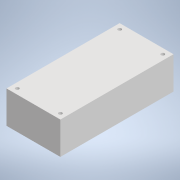
# Autodesk Inventor part: LPS_board
Saved by Autodesk Inventor 2022 (Build 260153000, 153)
## iProperties
Created: 2024-07-06
Part Number: LPS_board
Material: Типовые
Document SubType Name: Modeling
Designer: Капустяник Андрей
Density: 1 g/cm^3
Appearance: По умолчанию
Author: Капустяник Андрей
Autodesk Inventor part; units mm, degrees
ref_plane "YZ Plane" through (0, 0, 0) normal (1, 0, 0) x (0, 1, 0)
ref_plane "XZ Plane" through (0, 0, 0) normal (0, 1, 0) x (-1, 0, 0)
ref_plane "XY Plane" through (0, 0, 0) normal (0, 0, 1) x (1, 0, 0)
sketch "Эскиз1" plane through (0, 0, 0) normal (0, 1, 0) x (-1, 0, 0)
  line L0 (-25, 52.5) -> (25, 52.5)
  line L1 (25, 52.5) -> (25, -52.5)
  line L2 (25, -52.5) -> (-25, -52.5)
  line L3 (-25, -52.5) -> (-25, 52.5)
  line L4 (-25, 52.5) -> (25, -52.5) construction
  line L5 (25, 52.5) -> (-25, -52.5) construction
  point P0 (0, 0)
  dimension "d0" = 50
  dimension "d1" = 105
  constraints: 12 end point, 2 midpoint, 2 parallel, 1 horizontal, 1 perpendicular
  measures "d0" distance of L1.end L2.end
  measures "d1" distance of L0.end L1.end
extrude "Выдавливание1" add sketch "Эскиз1" along normal blind 30
sketch "Эскиз2" plane through (0, 30, 0) normal (0, 1, 0) x (1, 0, 0)
  line L0 (25, 52.5) -> (-25, 52.5) projected
  line L1 (-25, 52.5) -> (-25, -52.5) projected
  line L2 (-25, -52.5) -> (25, -52.5) projected
  line L3 (25, -52.5) -> (25, 52.5) projected
  circle A0 centre (20, 47.5) radius 1.6
  circle A1 centre (20, -47.5) radius 1.6
  circle A2 centre (-20, -47.5) radius 1.6
  arc A3 (-20, 52.5) -> (-25, 47.5) centre (-20, 47.5) ccw projected
  circle A4 centre (-20, 47.5) radius 1.6
  point P0 (0, 0)
  dimension "d5" = 3.2
  dimension "d6" = 3.2
  dimension "d7" = 3.2
  dimension "d8" = 3.2
  constraints: 4 centre point, 1 coincident
  measures "d5" diameter of A0
  measures "d6" diameter of A1
  measures "d7" diameter of A2
  measures "d8" diameter of A4
extrude "Выдавливание2" cut sketch "Эскиз2" against normal blind 30 contours A0 | A1 | A2 | A4
